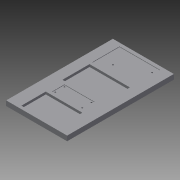
# Autodesk Inventor part: base embed
Saved by Autodesk Inventor 2015 (Build 190159000, 159)
## iProperties
Created: 2015-03-25
Part Number: base embed
Material: Generic
Document SubType Name: Modeling
Designer: Mitchell
Density: 1 g/cm^3
Appearance: Default
Author: Mitchell
Autodesk Inventor part; units mm, degrees
ref_plane "YZ Plane" through (0, 0, 0) normal (1, 0, 0) x (0, 1, 0)
ref_plane "XZ Plane" through (0, 0, 0) normal (0, 1, 0) x (-1, 0, 0)
ref_plane "XY Plane" through (0, 0, 0) normal (0, 0, 1) x (1, 0, 0)
sketch "Sketch1" plane through (0, 0, 0) normal (0, 1, 0) x (-1, 0, 0)
  line L0 (0, 0) -> (-127, 0)
  line L1 (-127, 0) -> (-127, -222.25)
  line L2 (-127, -222.25) -> (0, -222.25)
  line L3 (0, -222.25) -> (0, 0)
  line L4 (0, 0) -> (-25.4, 0)
  line L5 (-127, 0) -> (-101.6, 0)
  line L6 (-25.4, 0) -> (-25.4, -6.35)
  line L7 (-101.6, 0) -> (-101.6, -6.35)
  line L8 (-25.4, -6.35) -> (-101.6, -6.35)
  line L9 (-101.6, -6.35) -> (-101.6, -57.15)
  line L10 (-101.6, -57.15) -> (-25.4, -57.15)
  line L11 (-25.4, -57.15) -> (-25.4, -6.35)
  dimension "d0" = 222.25
  dimension "d1" = 127
  dimension "d2" = 25.4
  dimension "d3" = 25.4
  dimension "d4" = 6.35
  dimension "d5" = 6.35
  dimension "d6" = 50.8
  constraints: 24 end point, 4 parallel, 3 perpendicular, 2 horizontal, 2 point on line, 1 vertical
  measures "d0" distance of L1.end L0.end
  measures "d1" distance of L1.end L2.end
  measures "d2" distance of L0.start L4.end
  measures "d3" distance of L0.end L5.end
  measures "d4" distance of L4.end L6.end
  measures "d5" distance of L5.end L7.end
  measures "d6" distance of L9.end L8.end
extrude "Extrusion1" add sketch "Sketch1" along normal blind 10.16
sketch "Sketch3" plane through (0, 10.16, 0) normal (0, 1, 0) x (1, 0, 0)
  line L0 (0, 0) -> (25.4, 0)
  line L1 (0, 0) -> (127, 0) projected
  line L2 (25.4, 0) -> (25.4, 6.35)
  line L3 (127, 0) -> (101.6, 0)
  line L4 (101.6, 0) -> (101.6, 6.35)
  line L5 (25.4, 6.35) -> (101.6, 6.35)
  line L6 (101.6, 6.35) -> (101.6, 57.15)
  line L7 (101.6, 57.15) -> (25.4, 57.15)
  line L8 (25.4, 57.15) -> (25.4, 6.35)
  line L9 (0, 222.25) -> (0, 0) projected
  line L10 (0, 57.15) -> (31.9532, 57.15)
  line L11 (127, 57.15) -> (95.0468, 57.15)
  line L12 (31.9532, 57.15) -> (31.9532, 63.5)
  line L13 (95.0468, 57.15) -> (95.0468, 63.5)
  line L14 (31.9532, 63.5) -> (95.0468, 63.5)
  line L15 (95.0468, 63.5) -> (95.0468, 89.4842)
  line L16 (95.0468, 89.4842) -> (31.9532, 89.4842)
  line L17 (31.9532, 89.4842) -> (31.9532, 63.5)
  line L18 (31.9532, 63.5) -> (31.9532, 66.929)
  line L19 (31.9532, 66.929) -> (35.3822, 66.929)
  line L20 (31.9532, 89.4842) -> (31.9532, 86.0552)
  line L21 (31.9532, 86.0552) -> (35.3822, 86.0552)
  line L22 (95.0468, 63.5) -> (95.0468, 66.929)
  line L23 (95.0468, 66.929) -> (91.6178, 66.929)
  line L24 (95.0468, 89.4842) -> (95.0468, 86.0552)
  line L25 (95.0468, 86.0552) -> (91.6178, 86.0552)
  circle A0 centre (91.6178, 66.929) radius 1.4478
  circle A1 centre (91.6178, 86.0552) radius 1.4478
  circle A2 centre (35.3822, 66.929) radius 1.4478
  circle A3 centre (35.3822, 86.0552) radius 1.4478
  line L26 (0, 89.4842) -> (21.463, 89.4842)
  line L27 (127, 0) -> (127, 222.25) projected
  line L28 (127, 89.4842) -> (105.537, 89.4842)
  line L29 (21.463, 89.4842) -> (21.463, 95.8342)
  line L30 (105.537, 89.4842) -> (105.537, 95.8342)
  line L31 (21.463, 95.8342) -> (105.537, 95.8342)
  line L32 (105.537, 95.8342) -> (105.537, 152.2222)
  line L33 (105.537, 152.2222) -> (21.463, 152.2222)
  line L34 (21.463, 152.2222) -> (21.463, 95.8342)
  line L35 (0, 152.2222) -> (20.7518, 152.2222)
  line L36 (127, 152.2222) -> (106.2482, 152.2222)
  line L37 (106.2482, 152.2222) -> (106.2482, 158.5722)
  line L38 (20.7518, 152.2222) -> (20.7518, 158.5722)
  line L39 (20.7518, 158.5722) -> (105.537, 158.5722)
  line L40 (105.537, 158.5722) -> (105.537, 215.2904)
  line L41 (105.537, 215.2904) -> (20.7518, 215.2904)
  line L42 (20.7518, 215.2904) -> (20.7518, 158.5722)
  line L43 (20.7518, 158.5722) -> (20.7518, 176.5554)
  line L44 (20.7518, 176.5554) -> (46.0502, 176.5554)
  line L45 (105.537, 215.2904) -> (105.537, 203.0984)
  line L46 (105.537, 203.0984) -> (100.9142, 203.0984)
  circle A4 centre (46.0502, 176.5554) radius 1.5494
  circle A5 centre (100.9142, 203.0984) radius 1.5494
  dimension "d15" = 25.4
  dimension "d16" = 6.35
  dimension "d17" = 25.4
  dimension "d18" = 6.35
  dimension "d19" = 50.8
  dimension "d20" = 31.9532
  dimension "d21" = 31.9532
  dimension "d22" = 6.35
  dimension "d23" = 25.9842
  dimension "d24" = 3.429
  dimension "d25" = 3.429
  dimension "d26" = 3.429
  dimension "d27" = 3.429
  dimension "d28" = 2.8956
  dimension "d29" = 2.8956
  dimension "d30" = 2.8956
  dimension "d31" = 2.8956
  dimension "d32" = 21.463
  dimension "d33" = 21.463
  dimension "d34" = 6.35
  dimension "d35" = 6.35
  dimension "d36" = 56.388
  dimension "d37" = 20.7518
  dimension "d38" = 20.7518
  dimension "d39" = 6.35
  dimension "d40" = 56.7182
  dimension "d41" = 17.9832
  dimension "d42" = 25.2984
  dimension "d43" = 12.192
  dimension "d44" = 4.6228
  dimension "d45" = 3.0988
  dimension "d46" = 3.0988
  constraints: 88 end point, 19 point on line, 12 perpendicular, 8 parallel, 6 centre point, 6 coincident, 5 horizontal, 5 vertical
  measures "d15" distance of L0.start L0.end
  measures "d16" distance of L0.end L2.end
  measures "d17" distance of L1.end L3.end
  measures "d18" distance of L3.end L4.end
  measures "d19" distance of L6.end L5.end
  measures "d20" distance of L10.start L10.end
  measures "d21" distance of L11.start L11.end
  measures "d22" distance of L10.end L12.end
  measures "d23" distance of L15.end L14.end
  measures "d24" distance of L12.end L18.end
  measures "d25" distance of L18.end L19.end
  measures "d26" distance of L16.end L20.end
  measures "d27" distance of L22.end L23.end
  measures "d28" diameter of A0
  measures "d29" diameter of A1
  measures "d30" diameter of A2
  measures "d31" diameter of A3
  measures "d32" distance of L26.start L26.end
  measures "d33" distance of L28.start L28.end
  measures "d34" distance of L26.end L29.end
  measures "d35" distance of L28.end L30.end
  measures "d36" distance of L32.end L31.end
  measures "d37" distance of L35.start L35.end
  measures "d38" distance of L36.start L36.end
  measures "d39" distance of L36.end L37.end
  measures "d40" distance of L40.end L39.end
  measures "d41" distance of L38.end L43.end
  measures "d42" distance of L43.end L44.end
  measures "d43" distance of L40.end L45.end
  measures "d44" distance of L45.end L46.end
  measures "d45" diameter of A4
  measures "d46" diameter of A5
sketch "Sketch4" plane through (0, 10.16, 0) normal (0, 1, 0) x (1, 0, 0)
  circle A0 centre (91.6178, 66.929) radius 1.4478
  circle A1 centre (91.6178, 86.0552) radius 1.4478
  circle A2 centre (35.3822, 66.929) radius 1.4478
  circle A3 centre (35.3822, 86.0552) radius 1.4478
  circle A4 centre (46.0502, 176.5554) radius 1.5494
  circle A5 centre (100.9142, 203.0984) radius 1.5494
  point P0 (0, 0)
  dimension "d47" = 2.8956
  dimension "d48" = 2.8956
  dimension "d49" = 2.8956
  dimension "d50" = 2.8956
  dimension "d51" = 3.0988
  dimension "d52" = 3.0988
  constraints: 6 centre point
  measures "d47" diameter of A0
  measures "d48" diameter of A1
  measures "d49" diameter of A2
  measures "d50" diameter of A3
  measures "d51" diameter of A4
  measures "d52" diameter of A5
extrude "Extrusion2" cut sketch "Sketch3" against normal blind 5.08 contours L8 L7 L6 L5 | L34 L33 L32 L31
sketch "Sketch5" plane through (0, 10.16, 0) normal (0, 1, 0) x (1, 0, 0)
  line L0 (0, 0) -> (25.4, 0)
  line L1 (0, 0) -> (127, 0)
  line L2 (25.4, 0) -> (25.4, 6.35)
  line L3 (127, 0) -> (101.6, 0)
  line L4 (101.6, 0) -> (101.6, 6.35)
  line L5 (25.4, 6.35) -> (101.6, 6.35)
  line L6 (101.6, 6.35) -> (101.6, 57.15)
  line L7 (101.6, 57.15) -> (25.4, 57.15)
  line L8 (25.4, 57.15) -> (25.4, 6.35)
  line L9 (0, 222.25) -> (0, 0)
  line L10 (0, 57.15) -> (31.9532, 57.15)
  line L11 (127, 57.15) -> (95.0468, 57.15)
  line L12 (31.9532, 57.15) -> (31.9532, 63.5)
  line L13 (95.0468, 57.15) -> (95.0468, 63.5)
  line L14 (31.9532, 63.5) -> (95.0468, 63.5)
  line L15 (95.0468, 63.5) -> (95.0468, 89.4842)
  line L16 (95.0468, 89.4842) -> (31.9532, 89.4842)
  line L17 (31.9532, 89.4842) -> (31.9532, 63.5)
  line L18 (31.9532, 63.5) -> (31.9532, 66.929)
  line L19 (31.9532, 66.929) -> (35.3822, 66.929)
  line L20 (31.9532, 89.4842) -> (31.9532, 86.0552)
  line L21 (31.9532, 86.0552) -> (35.3822, 86.0552)
  line L22 (95.0468, 63.5) -> (95.0468, 66.929)
  line L23 (95.0468, 66.929) -> (91.6178, 66.929)
  line L24 (95.0468, 89.4842) -> (95.0468, 86.0552)
  line L25 (95.0468, 86.0552) -> (91.6178, 86.0552)
  circle A0 centre (91.6178, 66.929) radius 1.4478
  circle A1 centre (91.6178, 86.0552) radius 1.4478
  circle A2 centre (35.3822, 66.929) radius 1.4478
  circle A3 centre (35.3822, 86.0552) radius 1.4478
  line L26 (0, 89.4842) -> (21.463, 89.4842)
  line L27 (127, 0) -> (127, 222.25)
  line L28 (127, 89.4842) -> (105.537, 89.4842)
  line L29 (21.463, 89.4842) -> (21.463, 95.8342)
  line L30 (105.537, 89.4842) -> (105.537, 95.8342)
  line L31 (21.463, 95.8342) -> (105.537, 95.8342)
  line L32 (105.537, 95.8342) -> (105.537, 152.2222)
  line L33 (105.537, 152.2222) -> (21.463, 152.2222)
  line L34 (21.463, 152.2222) -> (21.463, 95.8342)
  line L35 (0, 152.2222) -> (20.7518, 152.2222)
  line L36 (127, 152.2222) -> (106.2482, 152.2222)
  line L37 (106.2482, 152.2222) -> (106.2482, 158.5722)
  line L38 (20.7518, 152.2222) -> (20.7518, 158.5722)
  line L39 (20.7518, 158.5722) -> (105.537, 158.5722)
  line L40 (105.537, 158.5722) -> (105.537, 215.2904)
  line L41 (105.537, 215.2904) -> (20.7518, 215.2904)
  line L42 (20.7518, 215.2904) -> (20.7518, 158.5722)
  line L43 (20.7518, 158.5722) -> (20.7518, 176.5554)
  line L44 (20.7518, 176.5554) -> (46.0502, 176.5554)
  line L45 (105.537, 215.2904) -> (105.537, 203.0984)
  line L46 (105.537, 203.0984) -> (100.9142, 203.0984)
  circle A4 centre (46.0502, 176.5554) radius 1.5494
  circle A5 centre (100.9142, 203.0984) radius 1.5494
  dimension "d55" = 25.4
  dimension "d56" = 6.35
  dimension "d57" = 25.4
  dimension "d58" = 6.35
  dimension "d59" = 50.8
  dimension "d60" = 31.9532
  dimension "d61" = 31.9532
  dimension "d62" = 6.35
  dimension "d63" = 25.9842
  dimension "d64" = 3.429
  dimension "d65" = 3.429
  dimension "d66" = 3.429
  dimension "d67" = 3.429
  dimension "d68" = 2.8956
  dimension "d69" = 2.8956
  dimension "d70" = 2.8956
  dimension "d71" = 2.8956
  dimension "d72" = 21.463
  dimension "d73" = 21.463
  dimension "d74" = 6.35
  dimension "d75" = 6.35
  dimension "d76" = 56.388
  dimension "d77" = 20.7518
  dimension "d78" = 20.7518
  dimension "d79" = 6.35
  dimension "d80" = 56.7182
  dimension "d81" = 17.9832
  dimension "d82" = 25.2984
  dimension "d83" = 12.192
  dimension "d84" = 4.6228
  dimension "d85" = 3.0988
  dimension "d86" = 3.0988
  constraints: 94 end point, 19 point on line, 12 perpendicular, 8 parallel, 6 centre point, 6 coincident, 5 horizontal, 5 vertical
  measures "d55" distance of L0.start L0.end
  measures "d56" distance of L0.end L2.end
  measures "d57" distance of L1.end L3.end
  measures "d58" distance of L3.end L4.end
  measures "d59" distance of L6.end L5.end
  measures "d60" distance of L10.start L10.end
  measures "d61" distance of L11.start L11.end
  measures "d62" distance of L10.end L12.end
  measures "d63" distance of L15.end L14.end
  measures "d64" distance of L12.end L18.end
  measures "d65" distance of L18.end L19.end
  measures "d66" distance of L16.end L20.end
  measures "d67" distance of L22.end L23.end
  measures "d68" diameter of A0
  measures "d69" diameter of A1
  measures "d70" diameter of A2
  measures "d71" diameter of A3
  measures "d72" distance of L26.start L26.end
  measures "d73" distance of L28.start L28.end
  measures "d74" distance of L26.end L29.end
  measures "d75" distance of L28.end L30.end
  measures "d76" distance of L32.end L31.end
  measures "d77" distance of L35.start L35.end
  measures "d78" distance of L36.start L36.end
  measures "d79" distance of L36.end L37.end
  measures "d80" distance of L40.end L39.end
  measures "d81" distance of L38.end L43.end
  measures "d82" distance of L43.end L44.end
  measures "d83" distance of L40.end L45.end
  measures "d84" distance of L45.end L46.end
  measures "d85" diameter of A4
  measures "d86" diameter of A5
extrude "Extrusion3" cut sketch "Sketch5" against normal blind 1.016 contours L42 L41 L40 L39 | L17 L16 L15 L14
extrude "Extrusion4" cut sketch "Sketch4" against normal blind 7.62
body "Solid1"
